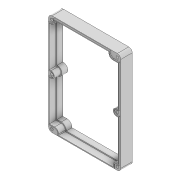
# Autodesk Inventor part: elektrobox EGI
Saved by Autodesk Inventor 2020.3 (Build 243373000, 373)
## iProperties
Created: 2020-12-12
Part Number: elektrobox EGI
Material: Generic
Document SubType Name: Modeling
Designer: Svend
Density: 1 g/cm^3
Appearance: Default
Author: Svend
Autodesk Inventor part; units mm, degrees
ref_plane "YZ Plane" through (0, 0, 0) normal (1, 0, 0) x (0, 1, 0)
ref_plane "XZ Plane" through (0, 0, 0) normal (0, 1, 0) x (-1, 0, 0)
ref_plane "XY Plane" through (0, 0, 0) normal (0, 0, 1) x (1, 0, 0)
sketch "Sketch1" plane through (0, 0, 0) normal (0, 0, 1) x (1, 0, 0)
  line L0 (-54.1322, 76.0214) -> (-53.917, 75.769)
  line L1 (40.9938, 75.769) -> (41.2072, 76.0214)
  line L2 (41.2072, 76.0214) -> (-54.1322, 76.0214)
  line L3 (-54.1322, 76.0214) -> (-54.1322, 72.8159)
  arc A0 (-59.6431, 67.3051) -> (-54.1322, 72.8159) centre (-59.6431, 72.8159) ccw
  line L4 (-59.6431, 67.3051) -> (-62.8486, 67.3051)
  line L5 (-62.8486, 67.3051) -> (-62.8486, -3.4861)
  line L6 (-62.8486, -3.4861) -> (-59.8427, -3.4861)
  arc A1 (-59.8427, -15.1085) -> (-59.8427, -3.4861) centre (-59.8427, -9.2973) ccw
  line L7 (-59.8427, -15.1085) -> (-62.8486, -15.1085)
  line L8 (-62.8486, -15.1085) -> (-62.8486, -85.5495)
  line L9 (-62.8486, -85.5495) -> (-53.6313, -85.5495)
  arc A2 (-46.6155, -92.5632) -> (-53.6313, -85.5495) centre (-53.6303, -92.5642) ccw
  line L10 (-46.6155, -92.5632) -> (-46.6155, -94.8177)
  line L11 (-46.4531, -94.5652) -> (-46.6155, -94.8177)
  line L12 (-46.6155, -94.8177) -> (48.673, -94.8177)
  line L13 (48.673, -94.8177) -> (48.4577, -94.5652)
  line L14 (55.9235, -91.1346) -> (55.9235, -93.5398)
  line L15 (55.9235, -93.5398) -> (53.5184, -93.5398)
  line L16 (53.5184, -93.5398) -> (53.5184, -91.1346)
  line L17 (53.5184, -91.1346) -> (55.9235, -91.1346)
  line L18 (53.5184, -10.8013) -> (53.5184, -8.3961)
  line L19 (53.5184, -8.3961) -> (55.9235, -8.3961)
  line L20 (55.9235, -8.3961) -> (55.9235, -10.8013)
  line L21 (55.9235, -10.8013) -> (53.5184, -10.8013)
  line L22 (55.9235, 74.3443) -> (55.9235, 71.9392)
  line L23 (55.9235, 71.9392) -> (53.5184, 71.9392)
  line L24 (53.5184, 71.9392) -> (53.5184, 74.3443)
  line L25 (53.5184, 74.3443) -> (55.9235, 74.3443)
  line L26 (-60.9816, 71.9392) -> (-60.9816, 74.3443)
  line L27 (-60.9816, 74.3443) -> (-58.5765, 74.3443)
  line L28 (-58.5765, 74.3443) -> (-58.5765, 71.9392)
  line L29 (-58.5765, 71.9392) -> (-60.9816, 71.9392)
  line L30 (-58.5765, -8.3961) -> (-58.5765, -10.8013)
  line L31 (-58.5765, -10.8013) -> (-60.9816, -10.8013)
  line L32 (-60.9816, -10.8013) -> (-60.9816, -8.3961)
  line L33 (-60.9816, -8.3961) -> (-58.5765, -8.3961)
  line L34 (-60.9816, -93.5398) -> (-60.9816, -91.1346)
  line L35 (-60.9816, -91.1346) -> (-58.5765, -91.1346)
  line L36 (-58.5765, -91.1346) -> (-58.5765, -93.5398)
  line L37 (-58.5765, -93.5398) -> (-60.9816, -93.5398)
  arc A3 (60.495, 73.0155) -> (54.4883, 79.0273) centre (54.4883, 73.0207) ccw
  line L38 (60.495, 73.0155) -> (60.495, -91.7609)
  arc A4 (54.4883, -97.7727) -> (60.495, -91.7609) centre (54.4883, -91.766) ccw
  line L39 (54.4883, -97.7727) -> (-59.5464, -97.7727)
  arc A5 (-65.5531, -91.7609) -> (-59.5464, -97.7727) centre (-59.5464, -91.766) ccw
  line L40 (-65.5531, -91.7609) -> (-65.5531, 73.0155)
  arc A6 (-59.5413, 79.0273) -> (-65.5531, 73.0155) centre (-59.5464, 73.0207) ccw
  line L41 (-59.5413, 79.0273) -> (54.4883, 79.0273)
  line L42 (-62.6979, -85.3244) -> (-53.4669, -85.3244)
  arc A7 (-46.4531, -92.3382) -> (-53.4669, -85.3244) centre (-53.462, -92.3333) ccw
  line L43 (-46.4531, -92.3382) -> (-46.4531, -94.5652)
  line L44 (-46.4531, -94.5652) -> (48.4577, -94.5652)
  line L45 (48.4577, -94.5652) -> (48.4577, -91.3362)
  arc A8 (53.9685, -85.8254) -> (48.4577, -91.3362) centre (53.9674, -91.3351) ccw
  line L46 (53.9685, -85.8254) -> (57.2386, -85.8254)
  line L47 (-62.6979, -3.2102) -> (-59.9542, -3.2102)
  arc A9 (-59.9542, -15.5841) -> (-59.9542, -3.2102) centre (-59.9532, -9.3971) ccw
  line L48 (-59.9542, -15.5841) -> (-62.6979, -15.5841)
  line L49 (57.2386, 66.5282) -> (48.0076, 66.5282)
  arc A10 (40.9938, 73.542) -> (48.0076, 66.5282) centre (48.0094, 73.5438) ccw
  line L50 (40.9938, 73.542) -> (40.9938, 75.769)
  line L51 (40.9938, 75.769) -> (-53.917, 75.769)
  line L52 (-53.917, 75.769) -> (-53.917, 72.54)
  arc A11 (-59.4278, 67.0292) -> (-53.917, 72.54) centre (-59.4299, 72.5421) ccw
  line L53 (-59.4278, 67.0292) -> (-62.6979, 67.0292)
  line L54 (57.2386, -15.6858) -> (54.5204, -15.6858)
  arc A12 (54.5204, -3.3609) -> (54.5204, -15.6858) centre (54.5204, -9.5234) ccw
  line L55 (54.5204, -3.3609) -> (57.2386, -3.3609)
  line L56 (36.348, -56.4885) -> (36.348, -54.1343)
  line L57 (36.348, -54.1343) -> (38.7022, -54.1343)
  line L58 (38.7022, -54.1343) -> (38.7022, -56.4885)
  line L59 (38.7022, -56.4885) -> (36.348, -56.4885)
  line L60 (-57.7879, -78.3107) -> (-57.7879, -75.9545)
  line L61 (-57.7879, -75.9545) -> (-55.4336, -75.9545)
  line L62 (-55.4336, -75.9545) -> (-55.4336, -78.3107)
  line L63 (-55.4336, -78.3107) -> (-57.7879, -78.3107)
  line L64 (-57.7879, -25.5039) -> (-57.7879, -23.1497)
  line L65 (-57.7879, -23.1497) -> (-55.4336, -23.1497)
  line L66 (-55.4336, -23.1497) -> (-55.4336, -25.5039)
  line L67 (-55.4336, -25.5039) -> (-57.7879, -25.5039)
  line L68 (-57.7879, 4.3554) -> (-57.7879, 6.7097)
  line L69 (-57.7879, 6.7097) -> (-55.4336, 6.7097)
  line L70 (-55.4336, 6.7097) -> (-55.4336, 4.3554)
  line L71 (-55.4336, 4.3554) -> (-57.7879, 4.3554)
  line L72 (-43.911, 35.7393) -> (-43.911, 38.0955)
  line L73 (-43.911, 38.0955) -> (-41.5568, 38.0955)
  line L74 (-41.5568, 38.0955) -> (-41.5568, 35.7393)
  line L75 (-41.5568, 35.7393) -> (-43.911, 35.7393)
  line L76 (-57.7879, 57.1602) -> (-57.7879, 59.5144)
  line L77 (-57.7879, 59.5144) -> (-55.4336, 59.5144)
  line L78 (-55.4336, 59.5144) -> (-55.4336, 57.1602)
  line L79 (-55.4336, 57.1602) -> (-57.7879, 57.1602)
  line L80 (52.3795, 57.1602) -> (50.0252, 57.1602)
  line L81 (50.0252, 57.1602) -> (50.0252, 59.5144)
  line L82 (50.0252, 59.5144) -> (52.3795, 59.5144)
  line L83 (52.3795, 59.5144) -> (52.3795, 57.1602)
  line L84 (36.348, 35.7393) -> (36.348, 38.0955)
  line L85 (36.348, 38.0955) -> (38.7022, 38.0955)
  line L86 (38.7022, 38.0955) -> (38.7022, 35.7393)
  line L87 (38.7022, 35.7393) -> (36.348, 35.7393)
  line L88 (50.0252, 4.3554) -> (50.0252, 6.7097)
  line L89 (50.0252, 6.7097) -> (52.3795, 6.7097)
  line L90 (52.3795, 6.7097) -> (52.3795, 4.3554)
  line L91 (52.3795, 4.3554) -> (50.0252, 4.3554)
  line L92 (50.0252, -25.5039) -> (50.0252, -23.1497)
  line L93 (50.0252, -23.1497) -> (52.3795, -23.1497)
  line L94 (52.3795, -23.1497) -> (52.3795, -25.5039)
  line L95 (52.3795, -25.5039) -> (50.0252, -25.5039)
  line L96 (-43.911, -56.4885) -> (-43.911, -54.1343)
  line L97 (-43.911, -54.1343) -> (-41.5568, -54.1343)
  line L98 (-41.5568, -54.1343) -> (-41.5568, -56.4885)
  line L99 (-41.5568, -56.4885) -> (-43.911, -56.4885)
  line L100 (50.0252, -78.3107) -> (50.0252, -75.9545)
  line L101 (50.0252, -75.9545) -> (52.3795, -75.9545)
  line L102 (52.3795, -75.9545) -> (52.3795, -78.3107)
  line L103 (52.3795, -78.3107) -> (50.0252, -78.3107)
  line L104 (-62.6979, -34.6723) -> (-62.6979, -59.7234)
  line L105 (-62.6979, -61.2264) -> (-62.6979, -64.0307)
  line L106 (-62.6979, -65.5336) -> (-62.6979, -85.3244)
  line L107 (-62.6979, -85.3244) -> (-62.8486, -85.5495)
  line L108 (-62.6979, -28.8621) -> (-62.6979, -15.5841)
  line L109 (-62.6979, -15.5841) -> (-62.8486, -15.1085)
  line L110 (-62.6979, -30.365) -> (-62.6979, -33.1694)
  line L111 (-62.6979, 13.923) -> (-62.6979, 11.1187)
  line L112 (-62.6979, 9.6158) -> (-62.6979, -3.2102)
  line L113 (-62.6979, -3.2102) -> (-62.8486, -3.4861)
  line L114 (-62.8486, 67.3051) -> (-62.6979, 67.0292)
  line L115 (-62.6979, 67.0292) -> (-62.6979, 46.2873)
  line L116 (-62.6979, 44.7844) -> (-62.6979, 41.98)
  line L117 (-62.6979, 40.4771) -> (-62.6979, 15.426)
  line L118 (-62.8251, -64.0307) -> (-61.2712, -64.0307)
  line L119 (-61.2712, -64.0307) -> (-61.146, -64.0307)
  line L120 (-61.146, -64.0307) -> (-61.146, -65.5336)
  line L121 (-61.146, -65.5336) -> (-61.2712, -65.5336)
  line L122 (-61.2712, -65.5336) -> (-62.8251, -65.5336)
  line L123 (-62.8251, -65.5336) -> (-62.8251, -64.0307)
  line L124 (-61.2712, -64.0307) -> (-61.2712, -65.5336)
  line L125 (-61.2712, 11.1187) -> (-61.146, 11.1187)
  line L126 (-61.146, 11.1187) -> (-61.146, 9.6158)
  line L127 (-61.146, 9.6158) -> (-61.2712, 9.6158)
  line L128 (-61.2712, 9.6158) -> (-62.8251, 9.6158)
  line L129 (-62.8251, 9.6158) -> (-62.8251, 11.1187)
  line L130 (-62.8251, 11.1187) -> (-61.2712, 11.1187)
  line L131 (-61.2712, 11.1187) -> (-61.2712, 9.6158)
  line L132 (-61.2712, 41.98) -> (-61.146, 41.98)
  line L133 (-61.146, 41.98) -> (-61.146, 40.4771)
  line L134 (-61.146, 40.4771) -> (-61.2712, 40.4771)
  line L135 (-61.2712, 40.4771) -> (-62.8251, 40.4771)
  line L136 (-62.8251, 40.4771) -> (-62.8251, 41.98)
  line L137 (-62.8251, 41.98) -> (-61.2712, 41.98)
  line L138 (-61.2712, 41.98) -> (-61.2712, 40.4771)
  line L139 (-61.2712, -28.8621) -> (-61.146, -28.8621)
  line L140 (-61.146, -28.8621) -> (-61.146, -30.365)
  line L141 (-61.146, -30.365) -> (-61.2712, -30.365)
  line L142 (-61.2712, -30.365) -> (-62.8251, -30.365)
  line L143 (-62.8251, -30.365) -> (-62.8251, -28.8621)
  line L144 (-62.8251, -28.8621) -> (-61.2712, -28.8621)
  line L145 (-61.2712, -28.8621) -> (-61.2712, -30.365)
  line L146 (-61.2712, -59.7234) -> (-61.146, -59.7234)
  line L147 (-61.146, -59.7234) -> (-61.146, -61.2264)
  line L148 (-61.146, -61.2264) -> (-61.2712, -61.2264)
  line L149 (-61.2712, -61.2264) -> (-62.8251, -61.2264)
  line L150 (-62.8251, -61.2264) -> (-62.8251, -59.7234)
  line L151 (-62.8251, -59.7234) -> (-61.2712, -59.7234)
  line L152 (-61.2712, -59.7234) -> (-61.2712, -61.2264)
  line L153 (-61.2712, 46.2873) -> (-61.146, 46.2873)
  line L154 (-61.146, 46.2873) -> (-61.146, 44.7844)
  line L155 (-61.146, 44.7844) -> (-61.2712, 44.7844)
  line L156 (-61.2712, 44.7844) -> (-62.8251, 44.7844)
  line L157 (-62.8251, 44.7844) -> (-62.8251, 46.2873)
  line L158 (-62.8251, 46.2873) -> (-61.2712, 46.2873)
  line L159 (-61.2712, 46.2873) -> (-61.2712, 44.7844)
  line L160 (-61.2712, 15.426) -> (-61.146, 15.426)
  line L161 (-61.146, 15.426) -> (-61.146, 13.923)
  line L162 (-61.146, 13.923) -> (-61.2712, 13.923)
  line L163 (-61.2712, 13.923) -> (-62.8251, 13.923)
  line L164 (-62.8251, 13.923) -> (-62.8251, 15.426)
  line L165 (-62.8251, 15.426) -> (-61.2712, 15.426)
  line L166 (-61.2712, 15.426) -> (-61.2712, 13.923)
  line L167 (-61.2712, -33.1694) -> (-61.146, -33.1694)
  line L168 (-61.146, -33.1694) -> (-61.146, -34.6723)
  line L169 (-61.146, -34.6723) -> (-61.2712, -34.6723)
  line L170 (-61.2712, -34.6723) -> (-62.8251, -34.6723)
  line L171 (-62.8251, -34.6723) -> (-62.8251, -33.1694)
  line L172 (-62.8251, -33.1694) -> (-61.2712, -33.1694)
  line L173 (-61.2712, -33.1694) -> (-61.2712, -34.6723)
  line L174 (57.2386, 11.2674) -> (57.2386, 14.0737)
  line L175 (57.2386, 15.5767) -> (57.2386, 40.6258)
  line L176 (57.2386, 42.1307) -> (57.2386, 44.935)
  line L177 (57.2386, 46.438) -> (57.2386, 66.5282)
  line L178 (57.2386, 66.5282) -> (57.3893, 66.7532)
  line L179 (57.2386, 9.7645) -> (57.2386, -3.3609)
  line L180 (57.2386, -3.3609) -> (57.3893, -3.5859)
  line L181 (57.2386, -28.6605) -> (57.2386, -15.6858)
  line L182 (57.2386, -15.6858) -> (57.3893, -15.2083)
  line L183 (57.2386, -65.334) -> (57.2386, -85.8254)
  line L184 (57.2386, -85.8254) -> (57.3893, -86.0505)
  line L185 (57.3893, -86.0505) -> (54.1838, -86.0505)
  arc A13 (54.1838, -86.0505) -> (48.673, -91.5613) centre (54.1838, -91.5613) ccw
  line L186 (48.673, -91.5613) -> (48.673, -94.8177)
  line L187 (57.2386, -63.8311) -> (57.2386, -61.0248)
  line L188 (57.2386, -59.5218) -> (57.2386, -34.4727)
  line L189 (57.2386, -32.9698) -> (57.2386, -30.1635)
  line L190 (57.3658, 44.935) -> (55.8629, 44.935)
  line L191 (55.8629, 44.935) -> (55.7357, 44.935)
  line L192 (55.7357, 44.935) -> (55.7357, 46.438)
  line L193 (55.7357, 46.438) -> (55.8629, 46.438)
  line L194 (55.8629, 46.438) -> (57.3658, 46.438)
  line L195 (57.3658, 46.438) -> (57.3658, 44.935)
  line L196 (55.8629, 44.935) -> (55.8629, 46.438)
  line L197 (55.8629, -34.4727) -> (55.7357, -34.4727)
  line L198 (55.7357, -34.4727) -> (55.7357, -32.9698)
  line L199 (55.7357, -32.9698) -> (55.8629, -32.9698)
  line L200 (55.8629, -32.9698) -> (57.3658, -32.9698)
  line L201 (57.3658, -32.9698) -> (57.3658, -34.4727)
  line L202 (57.3658, -34.4727) -> (55.8629, -34.4727)
  line L203 (55.8629, -34.4727) -> (55.8629, -32.9698)
  line L204 (55.8629, -65.334) -> (55.7357, -65.334)
  line L205 (55.7357, -65.334) -> (55.7357, -63.8311)
  line L206 (55.7357, -63.8311) -> (55.8629, -63.8311)
  line L207 (55.8629, -63.8311) -> (57.3658, -63.8311)
  line L208 (57.3658, -63.8311) -> (57.3658, -65.334)
  line L209 (57.3658, -65.334) -> (55.8629, -65.334)
  line L210 (55.8629, -65.334) -> (55.8629, -63.8311)
  line L211 (55.8629, 14.0737) -> (55.7357, 14.0737)
  line L212 (55.7357, 14.0737) -> (55.7357, 15.5767)
  line L213 (55.7357, 15.5767) -> (55.8629, 15.5767)
  line L214 (55.8629, 15.5767) -> (57.3658, 15.5767)
  line L215 (57.3658, 15.5767) -> (57.3658, 14.0737)
  line L216 (57.3658, 14.0737) -> (55.8629, 14.0737)
  line L217 (55.8629, 14.0737) -> (55.8629, 15.5767)
  line L218 (55.8629, 40.6258) -> (55.7357, 40.6258)
  line L219 (55.7357, 40.6258) -> (55.7357, 42.1307)
  line L220 (55.7357, 42.1307) -> (55.8629, 42.1307)
  line L221 (55.8629, 42.1307) -> (57.3658, 42.1307)
  line L222 (57.3658, 42.1307) -> (57.3658, 40.6258)
  line L223 (57.3658, 40.6258) -> (55.8629, 40.6258)
  line L224 (55.8629, 40.6258) -> (55.8629, 42.1307)
  circle A14 centre (-51.8573, -91.8108) radius 2.3807
  line L225 (55.8629, 9.7645) -> (55.7357, 9.7645)
  line L226 (55.7357, 9.7645) -> (55.7357, 11.2674)
  line L227 (55.7357, 11.2674) -> (55.8629, 11.2674)
  line L228 (55.8629, 11.2674) -> (57.3658, 11.2674)
  line L229 (57.3658, 11.2674) -> (57.3658, 9.7645)
  line L230 (57.3658, 9.7645) -> (55.8629, 9.7645)
  line L231 (55.8629, 9.7645) -> (55.8629, 11.2674)
  circle A15 centre (46.1279, 73.0674) radius 2.3807
  line L232 (55.8629, -61.0248) -> (55.7357, -61.0248)
  line L233 (55.7357, -61.0248) -> (55.7357, -59.5218)
  line L234 (55.7357, -59.5218) -> (55.8629, -59.5218)
  line L235 (55.8629, -59.5218) -> (57.3658, -59.5218)
  line L236 (57.3658, -59.5218) -> (57.3658, -61.0248)
  line L237 (57.3658, -61.0248) -> (55.8629, -61.0248)
  line L238 (55.8629, -61.0248) -> (55.8629, -59.5218)
  line L239 (55.8629, -30.1635) -> (55.7357, -30.1635)
  line L240 (55.7357, -30.1635) -> (55.7357, -28.6605)
  line L241 (55.7357, -28.6605) -> (55.8629, -28.6605)
  line L242 (55.8629, -28.6605) -> (57.3658, -28.6605)
  line L243 (57.3658, -28.6605) -> (57.3658, -30.1635)
  line L244 (57.3658, -30.1635) -> (55.8629, -30.1635)
  line L245 (55.8629, -30.1635) -> (55.8629, -28.6605)
  circle A16 centre (37.5251, -55.3114) radius 3.0303
  circle A17 centre (-56.6127, -77.1316) radius 3.0304
  circle A18 centre (-56.6127, -24.3268) radius 3.0303
  circle A19 centre (-56.6127, 5.5326) radius 3.0303
  circle A20 centre (-42.7339, 36.9184) radius 3.0303
  circle A21 centre (-56.6127, 58.3373) radius 3.0303
  circle A22 centre (51.2024, 58.3373) radius 3.0303
  circle A23 centre (37.5251, 36.9184) radius 3.0303
  circle A24 centre (51.2024, 5.5326) radius 3.0303
  circle A25 centre (51.2024, -24.3268) radius 3.0303
  line L246 (41.2072, 76.0214) -> (41.2052, 73.768)
  arc A26 (41.2052, 73.768) -> (48.2209, 66.7532) centre (48.2204, 73.7685) ccw
  line L247 (48.2209, 66.7532) -> (57.3893, 66.7532)
  line L248 (57.3893, 66.7532) -> (57.3893, -3.5859)
  line L249 (57.3893, -3.5859) -> (54.4832, -3.5859)
  arc A27 (54.4832, -3.5859) -> (54.4832, -15.2083) centre (54.4822, -9.3971) ccw
  line L250 (54.4832, -15.2083) -> (57.3893, -15.2083)
  line L251 (57.3893, -15.2083) -> (57.3893, -86.0505)
  arc A28 (-47.9734, -92.4233) -> (-49.5938, -88.595) centre (-51.8574, -91.8102) ccw
  arc A29 (-47.9698, -92.5632) -> (-47.9734, -92.4233) centre (-53.6728, -92.6423) ccw
  line L252 (-47.9698, -92.5632) -> (-47.9698, -96.1699)
  line L253 (-47.9698, -96.1699) -> (50.0252, -96.1699)
  line L254 (50.0252, -96.1699) -> (50.0252, -91.5603)
  arc A30 (54.1838, -87.4027) -> (50.0252, -91.5603) centre (54.1833, -91.5608) ccw
  line L255 (54.1838, -87.4027) -> (58.7416, -87.4027)
  line L256 (58.7416, -87.4027) -> (58.7416, -13.8561)
  line L257 (58.7416, -13.8561) -> (54.4832, -13.8561)
  arc A31 (54.4832, -4.9382) -> (54.4832, -13.8561) centre (54.4842, -9.3971) ccw
  line L258 (54.4832, -4.9382) -> (58.7416, -4.9382)
  line L259 (58.7416, -4.9382) -> (58.7416, 68.1055)
  line L260 (58.7416, 68.1055) -> (48.2209, 68.1055)
  arc A32 (44.535, 69.4712) -> (48.2209, 68.1055) centre (48.2231, 73.7684) ccw
  arc A33 (42.5597, 74.7204) -> (44.535, 69.4712) centre (46.1281, 73.0669) ccw
  circle A34 centre (-42.7339, -55.3114) radius 3.0303
  circle A35 centre (51.2024, -77.1316) radius 3.0304
  arc A36 (44.5353, 69.4718) -> (42.5594, 74.72) centre (46.1276, 73.0674) ccw
  line L261 (42.5594, 74.72) -> (42.5594, 77.3756)
  line L262 (42.5594, 77.3756) -> (-55.4845, 77.3756)
  line L263 (-55.4845, 77.3756) -> (-55.4845, 72.8159)
  arc A37 (-59.6431, 68.6574) -> (-55.4845, 72.8159) centre (-59.643, 72.8159) ccw
  line L264 (-59.6431, 68.6574) -> (-64.2008, 68.6574)
  line L265 (-64.2008, 68.6574) -> (-64.2008, -4.8384)
  line L266 (-64.2008, -4.8384) -> (-59.8427, -4.8384)
  arc A38 (-59.8427, -13.7563) -> (-59.8427, -4.8384) centre (-59.8436, -9.2973) ccw
  line L267 (-59.8427, -13.7563) -> (-64.2008, -13.7563)
  line L268 (-64.2008, -13.7563) -> (-64.2008, -86.9017)
  line L269 (-64.2008, -86.9017) -> (-53.6313, -86.9017)
  arc A39 (-49.5945, -88.5951) -> (-53.6313, -86.9017) centre (-53.6317, -92.5611) ccw
  arc A40 (-49.5945, -88.5951) -> (-47.9728, -92.4236) centre (-51.8575, -91.8114) ccw
  line L270 (-59.7781, 76.3463) -> (-59.7781, 69.9353)
  line L271 (-56.5726, 73.1408) -> (-62.9855, 73.1408)
  line L272 (54.72, 76.3463) -> (54.72, 69.9353)
  line L273 (57.9275, 73.1408) -> (51.5145, 73.1408)
  line L274 (-59.7781, -6.3922) -> (-59.7781, -12.8052)
  line L275 (-56.5726, -9.5977) -> (-62.9855, -9.5977)
  line L276 (54.72, -6.3922) -> (54.72, -12.8052)
  line L277 (57.9275, -9.5977) -> (51.5145, -9.5977)
  line L278 (54.72, -89.1307) -> (54.72, -95.5437)
  line L279 (57.9275, -92.3362) -> (51.5145, -92.3362)
  line L280 (-59.7781, -89.1307) -> (-59.7781, -95.5437)
  line L281 (-56.5726, -92.3362) -> (-62.9855, -92.3362)
  line L282 (46.1289, 79.0019) -> (46.1289, 67.129)
  line L283 (52.0644, 73.0664) -> (40.1915, 73.0664)
  line L284 (51.2014, 63.3716) -> (51.2014, 53.3011)
  line L285 (56.2366, 58.3363) -> (46.1661, 58.3363)
  line L286 (-51.8563, -85.8743) -> (-51.8563, -97.7472)
  line L287 (-45.9189, -91.8098) -> (-57.7918, -91.8098)
  line L288 (37.5241, 41.9526) -> (37.5241, 31.8821)
  line L289 (42.5594, 36.9174) -> (32.4908, 36.9174)
  line L290 (-42.7329, 41.9526) -> (-42.7329, 31.8821)
  line L291 (-37.6996, 36.9174) -> (-47.7682, 36.9174)
  line L292 (-56.6117, 63.3716) -> (-56.6117, 53.3011)
  line L293 (-51.5764, 58.3363) -> (-61.645, 58.3363)
  line L294 (-56.6117, 10.5668) -> (-56.6117, 0.4963)
  line L295 (-51.5764, 5.5316) -> (-61.645, 5.5316)
  line L296 (51.2014, 10.5668) -> (51.2014, 0.4963)
  line L297 (56.2366, 5.5316) -> (46.1661, 5.5316)
  line L298 (51.2014, -19.2925) -> (51.2014, -29.3611)
  line L299 (56.2366, -24.3278) -> (46.1661, -24.3278)
  line L300 (37.5241, -50.2771) -> (37.5241, -60.3457)
  line L301 (42.5594, -55.3105) -> (32.4908, -55.3105)
  line L302 (51.2014, -72.0973) -> (51.2014, -82.1659)
  line L303 (56.2366, -77.1306) -> (46.1661, -77.1306)
  line L304 (-56.6117, -72.0973) -> (-56.6117, -82.1659)
  line L305 (-51.5764, -77.1306) -> (-61.645, -77.1306)
  line L306 (-42.7329, -50.2771) -> (-42.7329, -60.3457)
  line L307 (-37.6996, -55.3105) -> (-47.7682, -55.3105)
  line L308 (-56.6117, -19.2925) -> (-56.6117, -29.3611)
  line L309 (-51.5764, -24.3278) -> (-61.645, -24.3278)
  line L310 (47.2052, -94.5633) -> (19.1639, -94.5633)
  line L311 (39.7414, 75.769) -> (19.1639, 75.769)
  line L312 (21.1678, -94.5633) -> (21.1678, -91.5574)
  line L313 (21.1678, -91.5574) -> (21.1678, 72.7631)
  line L314 (21.1678, 72.7631) -> (21.1678, 75.769)
  line L315 (21.9721, -91.5574) -> (21.1678, -94.5633)
  line L316 (21.1678, -94.5633) -> (20.3616, -91.5574)
  line L317 (20.3616, 72.7631) -> (21.1678, 75.769)
  line L318 (21.1678, 75.769) -> (21.9721, 72.7631)
  line L319 (-62.6979, -84.07) -> (-62.6979, -64.4514)
  line L320 (57.2386, -84.571) -> (57.2386, -64.4514)
  line L321 (-62.6979, -66.4554) -> (-59.692, -66.4554)
  line L322 (-59.692, -66.4554) -> (54.2327, -66.4554)
  line L323 (54.2327, -66.4554) -> (57.2386, -66.4554)
  line L324 (-59.692, -67.2616) -> (-62.6979, -66.4554)
  line L325 (-62.6979, -66.4554) -> (-59.692, -65.6511)
  line L326 (54.2327, -65.6511) -> (57.2386, -66.4554)
  line L327 (57.2386, -66.4554) -> (54.2327, -67.2616)
  line L328 (46.1289, -49.5002) -> (46.1289, -69.5395)
  line L329 (46.1289, -69.5395) -> (48.6651, -69.5395)
  line L330 (48.6651, -69.5395) -> (51.2014, -69.5395)
  line L331 (51.2014, -69.5395) -> (51.2014, -76.4789)
  line L332 (51.2014, -76.4789) -> (51.2014, -83.4183)
  line L333 (51.2014, -83.4183) -> (52.9607, -83.4183)
  line L334 (52.9607, -83.4183) -> (54.72, -83.4183)
  line L335 (54.72, -83.4183) -> (54.72, -103.4577)
  circle A41 centre (57.2376, 43.5329) radius 6.2378
  line L336 (-0.8402, 73.0664) -> (40.943, 73.0664)
  line L337 (40.943, 73.0664) -> (-0.8402, 73.0664)
  line L338 (-58.2888, 79.0273) -> (3.1677, 79.0273)
  line L339 (1.9681, 82.0332) -> (1.1637, 79.0273)
  line L340 (1.1637, 79.0273) -> (0.3575, 82.0332)
  line L341 (-54.5354, -91.8098) -> (3.1677, -91.8098)
  line L342 (1.1637, 73.0664) -> (1.1637, 70.0605)
  line L343 (1.1637, 70.0605) -> (1.1637, -88.8039)
  line L344 (1.1637, -88.8039) -> (1.1637, -91.8098)
  line L345 (1.9681, -88.8039) -> (1.1637, -91.8098)
  line L346 (1.1637, -91.8098) -> (0.3575, -88.8039)
  line L347 (-29.6976, 61.8413) -> (-51.414, 69.6554)
  line L348 (-51.414, 69.6554) -> (-54.2418, 70.673)
  line L349 (-54.2418, 70.673) -> (-51.142, 70.4128)
  line L350 (-59.4278, 72.54) -> (-54.2418, 70.673)
  line L351 (-54.2418, 70.673) -> (-51.686, 68.8981)
  line L352 (27.8039, 63.3266) -> (39.0662, 69.0194)
  line L353 (39.0662, 69.0194) -> (41.7473, 70.3775)
  line L354 (41.7473, 70.3775) -> (39.4283, 68.3012)
  line L355 (48.0076, 73.542) -> (41.7473, 70.3775)
  line L356 (41.7473, 70.3775) -> (38.7022, 69.7396)
  line L357 (-37.4393, -76.3459) -> (-46.3729, -85.2598)
  line L358 (-46.3729, -85.2598) -> (-48.5021, -87.3831)
  line L359 (-48.5021, -87.3831) -> (-46.9424, -84.6884)
  line L360 (-53.4669, -92.3362) -> (-48.5021, -87.3831)
  line L361 (-48.5021, -87.3831) -> (-45.8054, -85.8293)
  line L362 (30.5554, -79.342) -> (46.3892, -87.4516)
  line L363 (46.3892, -87.4516) -> (49.0644, -88.8215)
  line L364 (49.0644, -88.8215) -> (46.0213, -88.1679)
  line L365 (53.9685, -91.3343) -> (49.0644, -88.8215)
  line L366 (49.0644, -88.8215) -> (46.7551, -86.7354)
  line L367 (-53.7643, -8.1457) -> (-53.7643, 2.5002)
  line L368 (48.3559, -8.2709) -> (48.3559, 2.5002)
  line L369 (-53.7643, 0.4963) -> (-50.7584, 0.4963)
  line L370 (-50.7584, 0.4963) -> (45.35, 0.4963)
  line L371 (45.35, 0.4963) -> (48.3559, 0.4963)
  line L372 (-50.7584, -0.308) -> (-53.7643, 0.4963)
  line L373 (-53.7643, 0.4963) -> (-50.7584, 1.3026)
  line L374 (45.35, 1.3026) -> (48.3559, 0.4963)
  line L375 (48.3559, 0.4963) -> (45.35, -0.308)
  point P0 (-17.5057, 1.7531)
  point P1 (-22.7014, -65.1985)
  point P2 (-0.0931, -21.271)
  point P3 (19.913, -16.4667)
  point P4 (-42.4594, 67.7678)
  point P5 (27.9233, 64.7904)
  point P6 (-44.5862, -81.706)
  point P7 (31.8111, -78.5747)
  point P8 (-49.667, -88.5453)
  point P9 (-49.6555, -88.5339)
  point P10 (57.3893, 49.7689)
  point P11 (58.7416, 49.5867)
  point P12 (58.7416, 37.4791)
  point P13 (57.3893, 37.2969)
  dimension "d3" = 176.8
  constraints: 752 end point, 64 point on line, 54 point on circle, 42 centre point, 8 other
  measures "d3" distance between parallel lines of L39 L338
extrude "Extrusion1" add sketch "Sketch1" along normal blind 20 contours L3 A0 L350 A37 L263 L262 L261 A33 L283 A26 L246 L2 | A0 L4 L5 L6 A1 L7 L8 L9 A2 L360 A39 L269 L268 L267 A38 L266 L265 L264 A37 L350 | L283 A33 L355 A26 | A37 L264 L265 L266 A38 L267 L268 L269 A39 L286 A40 A29 L252 L253 L254 A30 L365 L17 L16 L15 L278 L335 A4 L39 A5 L40 A6 L41 A3 L38 A41 L259 L260 A32 L282 A36 L261 L262 L263 | L355 A33 A32 L260 L259 A41 L248 L247 A26 | L283 A15 L355 A33 | A33 A36 L282 A15 L283 | L355 A15 L282 A36 A33 | L283 L282 L355 A15 | A15 L282 L283 | A36 L282 A32 | L355 L282 A15 | A36 L283 A15 L282 | A15 L283 L282 | L283 L355 L282 | A41 L259 L248 | L282 A15 L283 A36 | L282 L355 L283 A15 | A41 L259 L258 A31 L257 L256 L255 L335 L185 L251 L250 A27 L249 L248 | A41 L38 L259 | A41 L38 A4 L335 L278 L15 L14 L17 L255 L256 L257 A31 L258 L259 | A2 L287 A28 A39 L360 | L12 L186 A13 L365 A30 L254 L253 L252 A29 A28 L287 A2 L10 | L360 A40 L286 A39 | L287 A14 L360 A40 A28 | A28 A40 L286 A14 L287 | L360 A14 L286 A40 | L286 A14 L287 A40 | A13 L185 L335 L255 A30 L365 | L287 L286 L360 A14 | A14 L286 L287 | L360 L286 A14 | L287 A14 L286 A40 | L286 L360 L287 A14 | A30 L255 L335 L278 L17 L365 | A14 L287 L286 | L287 L360 L286
sketch "Sketch2" plane through (0, 0, 20) normal (0, 0, 1) x (1, 0, 0)
  arc A0 (60.495, 73.0155) -> (54.4883, 79.0273) centre (54.4883, 73.0207) ccw projected
  line L0 (54.4883, 79.0273) -> (-59.5413, 79.0273) projected
  arc A1 (-59.5413, 79.0273) -> (-65.5531, 73.0155) centre (-59.5464, 73.0207) ccw projected
  line L1 (-65.5531, 73.0155) -> (-65.5531, -91.7609) projected
  arc A2 (-65.5531, -91.7609) -> (-59.5464, -97.7727) centre (-59.5464, -91.766) ccw projected
  line L2 (-59.5464, -97.7727) -> (54.4883, -97.7727) projected
  arc A3 (54.4883, -97.7727) -> (60.495, -91.7609) centre (54.4883, -91.766) ccw projected
  line L3 (60.495, -91.7609) -> (60.495, 73.0155) projected
  line L4 (-49.667, -88.5453) -> (-49.6555, -88.5339) projected
  arc A4 (-49.5945, -88.5951) -> (-49.6555, -88.5339) centre (-53.6317, -92.5611) ccw projected
  arc A5 (-49.5945, -88.5951) -> (-49.667, -88.5453) centre (-51.8575, -91.8114) ccw projected
  arc A6 (-46.6155, -92.5632) -> (-53.6313, -85.5495) centre (-53.6303, -92.5642) ccw projected
  line L5 (-53.6313, -85.5495) -> (-62.8486, -85.5495) projected
  line L6 (-62.8486, -85.5495) -> (-62.8486, -15.1085) projected
  line L7 (-62.8486, -15.1085) -> (-59.8427, -15.1085) projected
  arc A7 (-59.8427, -15.1085) -> (-59.8427, -3.4861) centre (-59.8427, -9.2973) ccw projected
  line L8 (-59.8427, -3.4861) -> (-62.8486, -3.4861) projected
  line L9 (-62.8486, -3.4861) -> (-62.8486, 67.3051) projected
  line L10 (-62.8486, 67.3051) -> (-59.6431, 67.3051) projected
  arc A8 (-59.6431, 67.3051) -> (-54.1322, 72.8159) centre (-59.6431, 72.8159) ccw projected
  line L11 (-54.1322, 72.8159) -> (-54.1322, 76.0214) projected
  line L12 (-54.1322, 76.0214) -> (41.2072, 76.0214) projected
  line L13 (41.2072, 76.0214) -> (41.2052, 73.768) projected
  arc A9 (41.2052, 73.768) -> (48.2209, 66.7532) centre (48.2204, 73.7685) ccw projected
  line L14 (48.2209, 66.7532) -> (57.3893, 66.7532) projected
  line L15 (57.3893, 66.7532) -> (57.3893, -3.5859) projected
  line L16 (57.3893, -3.5859) -> (54.4832, -3.5859) projected
  arc A10 (54.4832, -3.5859) -> (54.4832, -15.2083) centre (54.4822, -9.3971) ccw projected
  line L17 (54.4832, -15.2083) -> (57.3893, -15.2083) projected
  line L18 (57.3893, -15.2083) -> (57.3893, -86.0505) projected
  line L19 (57.3893, -86.0505) -> (54.1838, -86.0505) projected
  arc A11 (54.1838, -86.0505) -> (48.673, -91.5613) centre (54.1838, -91.5613) ccw projected
  line L20 (48.673, -91.5613) -> (48.673, -94.8177) projected
  line L21 (48.673, -94.8177) -> (-46.6155, -94.8177) projected
  line L22 (-46.6155, -94.8177) -> (-46.6155, -92.5632) projected
  line L23 (-58.5765, 74.3443) -> (-58.5765, 71.9392) projected
  line L24 (-58.5765, 71.9392) -> (-60.9816, 71.9392) projected
  line L25 (-60.9816, 71.9392) -> (-60.9816, 74.3443) projected
  line L26 (-60.9816, 74.3443) -> (-58.5765, 74.3443) projected
  line L27 (55.9235, -10.8013) -> (53.5184, -10.8013) projected
  line L28 (53.5184, -10.8013) -> (53.5184, -8.3961) projected
  line L29 (53.5184, -8.3961) -> (55.9235, -8.3961) projected
  line L30 (55.9235, -8.3961) -> (55.9235, -10.8013) projected
  line L31 (53.5184, 74.3443) -> (55.9235, 74.3443) projected
  line L32 (55.9235, 74.3443) -> (55.9235, 71.9392) projected
  line L33 (55.9235, 71.9392) -> (53.5184, 71.9392) projected
  line L34 (53.5184, 71.9392) -> (53.5184, 74.3443) projected
  line L35 (-60.9816, -8.3961) -> (-58.5765, -8.3961) projected
  line L36 (-58.5765, -8.3961) -> (-58.5765, -10.8013) projected
  line L37 (-58.5765, -10.8013) -> (-60.9816, -10.8013) projected
  line L38 (-60.9816, -10.8013) -> (-60.9816, -8.3961) projected
  line L39 (-58.5765, -93.5398) -> (-60.9816, -93.5398) projected
  line L40 (-60.9816, -93.5398) -> (-60.9816, -91.1346) projected
  line L41 (-60.9816, -91.1346) -> (-58.5765, -91.1346) projected
  line L42 (-58.5765, -91.1346) -> (-58.5765, -93.5398) projected
  line L43 (53.5184, -91.1346) -> (55.9235, -91.1346) projected
  line L44 (55.9235, -91.1346) -> (55.9235, -93.5398) projected
  line L45 (55.9235, -93.5398) -> (53.5184, -93.5398) projected
  line L46 (53.5184, -93.5398) -> (53.5184, -91.1346) projected
  line L47 (58.8893, 68.2532) -> (48.2204, 68.2532)
  arc A12 (42.7052, 73.7733) -> (48.2204, 68.2532) centre (48.2204, 73.7685) ccw
  line L48 (42.7052, 73.7733) -> (42.7085, 77.5214)
  line L49 (42.7085, 77.5214) -> (-55.6322, 77.5214)
  line L50 (-55.6322, 77.5214) -> (-55.6322, 72.8159)
  arc A13 (-59.6431, 68.8051) -> (-55.6322, 72.8159) centre (-59.6431, 72.8159) ccw
  line L51 (-59.6431, 68.8051) -> (-64.3486, 68.8051)
  line L52 (-64.3486, 68.8051) -> (-64.3486, -4.9861)
  line L53 (-64.3486, -4.9861) -> (-59.8427, -4.9861)
  arc A14 (-59.8427, -13.6085) -> (-59.8427, -4.9861) centre (-59.8427, -9.2973) ccw
  line L54 (-59.8427, -13.6085) -> (-64.3486, -13.6085)
  line L55 (-64.3486, -13.6085) -> (-64.3486, -87.0495)
  line L56 (-64.3486, -87.0495) -> (-53.6303, -87.0495)
  arc A15 (-48.1155, -92.5642) -> (-53.6303, -87.0495) centre (-53.6303, -92.5642) ccw
  line L57 (-48.1155, -92.5642) -> (-48.1155, -96.3177)
  line L58 (-48.1155, -96.3177) -> (50.173, -96.3177)
  line L59 (50.173, -96.3177) -> (50.173, -91.5613)
  arc A16 (54.1838, -87.5505) -> (50.173, -91.5613) centre (54.1838, -91.5613) ccw
  line L60 (54.1838, -87.5505) -> (58.8893, -87.5505)
  line L61 (58.8893, -87.5505) -> (58.8893, -13.7083)
  line L62 (58.8893, -13.7083) -> (54.4822, -13.7083)
  arc A17 (54.4822, -5.0859) -> (54.4822, -13.7083) centre (54.4822, -9.3971) ccw
  line L63 (54.4822, -5.0859) -> (58.8893, -5.0859)
  line L64 (58.8893, -5.0859) -> (58.8893, 68.2532)
  point P0 (0, 0)
  dimension "d4" = 1.5
  constraints: 36 end point, 12 point on circle, 6 centre point, 23 other
  measures "d4" distance between parallel lines of L14 L47
extrude "Extrusion2" add sketch "Sketch2" along normal blind 1.5 contours L64 L63 A17 L62 L61 L60 A16 L59 L58 L57 A15 L56 L55 L54 A14 L53 L52 L51 A13 L50 L49 L48 A12 L47
sketch "Sketch3" plane through (0, 0, 0) normal (0, 0, -1) x (-1, 0, 0)
  arc A0 (-54.4883, 79.0273) -> (-60.495, 73.0155) centre (-54.4883, 73.0207) ccw projected
  line L0 (-60.495, -91.7609) -> (-60.495, 73.0155) projected
  arc A1 (-60.495, -91.7609) -> (-54.4883, -97.7727) centre (-54.4883, -91.766) ccw projected
  line L1 (59.5464, -97.7727) -> (-54.4883, -97.7727) projected
  arc A2 (59.5464, -97.7727) -> (65.5531, -91.7609) centre (59.5464, -91.766) ccw projected
  line L2 (65.5531, 73.0155) -> (65.5531, -91.7609) projected
  arc A3 (65.5531, 73.0155) -> (59.5413, 79.0273) centre (59.5464, 73.0207) ccw projected
  line L3 (-54.4883, 79.0273) -> (59.5413, 79.0273) projected
  line L4 (49.667, -88.5453) -> (49.6555, -88.5339) projected
  arc A4 (49.667, -88.5453) -> (49.5945, -88.5951) centre (51.8575, -91.8114) ccw projected
  arc A5 (49.6555, -88.5339) -> (49.5945, -88.5951) centre (53.6317, -92.5611) ccw projected
  arc A6 (53.6313, -85.5495) -> (46.6155, -92.5632) centre (53.6303, -92.5642) ccw projected
  line L5 (46.6155, -94.8177) -> (46.6155, -92.5632) projected
  line L6 (-48.673, -94.8177) -> (46.6155, -94.8177) projected
  line L7 (-48.673, -91.5613) -> (-48.673, -94.8177) projected
  arc A7 (-48.673, -91.5613) -> (-54.1838, -86.0505) centre (-54.1838, -91.5613) ccw projected
  line L8 (-57.3893, -86.0505) -> (-54.1838, -86.0505) projected
  line L9 (-57.3893, -15.2083) -> (-57.3893, -86.0505) projected
  line L10 (-54.4832, -15.2083) -> (-57.3893, -15.2083) projected
  arc A8 (-54.4832, -15.2083) -> (-54.4832, -3.5859) centre (-54.4822, -9.3971) ccw projected
  line L11 (-57.3893, -3.5859) -> (-54.4832, -3.5859) projected
  line L12 (-57.3893, 66.7532) -> (-57.3893, -3.5859) projected
  line L13 (-48.2209, 66.7532) -> (-57.3893, 66.7532) projected
  arc A9 (-48.2209, 66.7532) -> (-41.2052, 73.768) centre (-48.2204, 73.7685) ccw projected
  line L14 (-41.2072, 76.0214) -> (-41.2052, 73.768) projected
  line L15 (54.1322, 76.0214) -> (-41.2072, 76.0214) projected
  line L16 (54.1322, 72.8159) -> (54.1322, 76.0214) projected
  arc A10 (54.1322, 72.8159) -> (59.6431, 67.3051) centre (59.6431, 72.8159) ccw projected
  line L17 (62.8486, 67.3051) -> (59.6431, 67.3051) projected
  line L18 (62.8486, -3.4861) -> (62.8486, 67.3051) projected
  line L19 (59.8427, -3.4861) -> (62.8486, -3.4861) projected
  arc A11 (59.8427, -3.4861) -> (59.8427, -15.1085) centre (59.8427, -9.2973) ccw projected
  line L20 (62.8486, -15.1085) -> (59.8427, -15.1085) projected
  line L21 (62.8486, -85.5495) -> (62.8486, -15.1085) projected
  line L22 (53.6313, -85.5495) -> (62.8486, -85.5495) projected
  line L23 (58.5765, 74.3443) -> (58.5765, 71.9392) projected
  line L24 (60.9816, 74.3443) -> (58.5765, 74.3443) projected
  line L25 (60.9816, 71.9392) -> (60.9816, 74.3443) projected
  line L26 (58.5765, 71.9392) -> (60.9816, 71.9392) projected
  line L27 (-55.9235, -10.8013) -> (-53.5184, -10.8013) projected
  line L28 (-55.9235, -8.3961) -> (-55.9235, -10.8013) projected
  line L29 (-53.5184, -8.3961) -> (-55.9235, -8.3961) projected
  line L30 (-53.5184, -10.8013) -> (-53.5184, -8.3961) projected
  line L31 (-53.5184, 74.3443) -> (-55.9235, 74.3443) projected
  line L32 (-53.5184, 71.9392) -> (-53.5184, 74.3443) projected
  line L33 (-55.9235, 71.9392) -> (-53.5184, 71.9392) projected
  line L34 (-55.9235, 74.3443) -> (-55.9235, 71.9392) projected
  line L35 (60.9816, -8.3961) -> (58.5765, -8.3961) projected
  line L36 (60.9816, -10.8013) -> (60.9816, -8.3961) projected
  line L37 (58.5765, -10.8013) -> (60.9816, -10.8013) projected
  line L38 (58.5765, -8.3961) -> (58.5765, -10.8013) projected
  line L39 (58.5765, -93.5398) -> (60.9816, -93.5398) projected
  line L40 (58.5765, -91.1346) -> (58.5765, -93.5398) projected
  line L41 (60.9816, -91.1346) -> (58.5765, -91.1346) projected
  line L42 (60.9816, -93.5398) -> (60.9816, -91.1346) projected
  line L43 (-53.5184, -91.1346) -> (-55.9235, -91.1346) projected
  line L44 (-53.5184, -93.5398) -> (-53.5184, -91.1346) projected
  line L45 (-55.9235, -93.5398) -> (-53.5184, -93.5398) projected
  line L46 (-55.9235, -91.1346) -> (-55.9235, -93.5398) projected
  arc A12 (-55.495, -17.0358) -> (-55.495, -1.7585) centre (-54.4822, -9.3971) ccw
  line L47 (-55.495, -17.0358) -> (-55.495, -84.2732)
  arc A13 (-46.905, -92.9234) -> (-55.495, -84.2732) centre (-54.1838, -91.5613) ccw
  line L48 (-46.905, -92.9234) -> (44.7285, -92.9234)
  arc A14 (53.6303, -83.6552) -> (44.7285, -92.9234) centre (53.6303, -92.5642) ccw
  line L49 (53.6303, -83.6552) -> (60.9543, -83.6552)
  line L50 (60.9543, -83.6552) -> (60.9543, -16.9222)
  arc A15 (60.9543, -1.6724) -> (60.9543, -16.9222) centre (59.8427, -9.2973) ccw
  line L51 (60.9543, -1.6724) -> (60.9543, 65.5278)
  arc A16 (52.355, 74.1271) -> (60.9543, 65.5278) centre (59.6431, 72.8159) ccw
  line L52 (52.355, 74.1271) -> (-39.3181, 74.1271)
  arc A17 (-48.2204, 64.8589) -> (-39.3181, 74.1271) centre (-48.2204, 73.7685) ccw
  line L53 (-48.2204, 64.8589) -> (-55.495, 64.8589)
  line L54 (-55.495, 64.8589) -> (-55.495, -1.7585)
  point P0 (0, 0)
  dimension "d7" = 5
  constraints: 16 end point, 12 point on circle, 6 centre point, 13 other
  measures "d7" distance between parallel lines of L0 L54
extrude "Extrusion3" add sketch "Sketch3" against normal blind 10 contours A6 L5 L6 L7 A7 L8 L9 L10 A8 L11 L12 L13 A9 L14 L15 L16 A10 L17 L18 L19 A11 L20 L21 L22
sketch "Sketch4" plane through (0, 0, 0) normal (0, 0, -1) x (-1, 0, 0)
  arc A0 (-46.905, -92.9234) -> (-55.495, -84.2732) centre (-54.1838, -91.5613) ccw projected
  line L0 (-55.495, -84.2732) -> (-55.495, -17.0358) projected
  arc A1 (-55.495, -17.0358) -> (-55.495, -1.7585) centre (-54.4822, -9.3971) ccw projected
  line L1 (-55.495, -1.7585) -> (-55.495, 64.8589) projected
  line L2 (-55.495, 64.8589) -> (-48.2204, 64.8589) projected
  arc A2 (-48.2204, 64.8589) -> (-39.3181, 74.1271) centre (-48.2204, 73.7685) ccw projected
  line L3 (-39.3181, 74.1271) -> (52.355, 74.1271) projected
  arc A3 (52.355, 74.1271) -> (60.9543, 65.5278) centre (59.6431, 72.8159) ccw projected
  line L4 (60.9543, 65.5278) -> (60.9543, -1.6724) projected
  arc A4 (60.9543, -1.6724) -> (60.9543, -16.9222) centre (59.8427, -9.2973) ccw projected
  line L5 (60.9543, -16.9222) -> (60.9543, -83.6552) projected
  line L6 (60.9543, -83.6552) -> (53.6303, -83.6552) projected
  arc A5 (53.6303, -83.6552) -> (44.7285, -92.9234) centre (53.6303, -92.5642) ccw projected
  line L7 (44.7285, -92.9234) -> (-46.905, -92.9234) projected
  arc A6 (-54.4883, 79.0273) -> (-60.495, 73.0155) centre (-54.4883, 73.0207) ccw projected
  line L8 (-60.495, -91.7609) -> (-60.495, 73.0155) projected
  arc A7 (-60.495, -91.7609) -> (-54.4883, -97.7727) centre (-54.4883, -91.766) ccw projected
  line L9 (59.5464, -97.7727) -> (-54.4883, -97.7727) projected
  arc A8 (59.5464, -97.7727) -> (65.5531, -91.7609) centre (59.5464, -91.766) ccw projected
  line L10 (65.5531, 73.0155) -> (65.5531, -91.7609) projected
  arc A9 (65.5531, 73.0155) -> (59.5413, 79.0273) centre (59.5464, 73.0207) ccw projected
  line L11 (-54.4883, 79.0273) -> (59.5413, 79.0273) projected
  line L12 (49.667, -88.5453) -> (49.6555, -88.5339) projected
  arc A10 (49.667, -88.5453) -> (49.5945, -88.5951) centre (51.8575, -91.8114) ccw projected
  arc A11 (49.6555, -88.5339) -> (49.5945, -88.5951) centre (53.6317, -92.5611) ccw projected
  line L13 (58.5765, 74.3443) -> (58.5765, 71.9392) projected
  line L14 (60.9816, 74.3443) -> (58.5765, 74.3443) projected
  line L15 (60.9816, 71.9392) -> (60.9816, 74.3443) projected
  line L16 (58.5765, 71.9392) -> (60.9816, 71.9392) projected
  line L17 (-55.9235, -10.8013) -> (-53.5184, -10.8013) projected
  line L18 (-55.9235, -8.3961) -> (-55.9235, -10.8013) projected
  line L19 (-53.5184, -8.3961) -> (-55.9235, -8.3961) projected
  line L20 (-53.5184, -10.8013) -> (-53.5184, -8.3961) projected
  line L21 (-53.5184, 74.3443) -> (-55.9235, 74.3443) projected
  line L22 (-53.5184, 71.9392) -> (-53.5184, 74.3443) projected
  line L23 (-55.9235, 71.9392) -> (-53.5184, 71.9392) projected
  line L24 (-55.9235, 74.3443) -> (-55.9235, 71.9392) projected
  line L25 (60.9816, -8.3961) -> (58.5765, -8.3961) projected
  line L26 (60.9816, -10.8013) -> (60.9816, -8.3961) projected
  line L27 (58.5765, -10.8013) -> (60.9816, -10.8013) projected
  line L28 (58.5765, -8.3961) -> (58.5765, -10.8013) projected
  line L29 (58.5765, -93.5398) -> (60.9816, -93.5398) projected
  line L30 (58.5765, -91.1346) -> (58.5765, -93.5398) projected
  line L31 (60.9816, -91.1346) -> (58.5765, -91.1346) projected
  line L32 (60.9816, -93.5398) -> (60.9816, -91.1346) projected
  line L33 (-53.5184, -91.1346) -> (-55.9235, -91.1346) projected
  line L34 (-53.5184, -93.5398) -> (-53.5184, -91.1346) projected
  line L35 (-55.9235, -93.5398) -> (-53.5184, -93.5398) projected
  line L36 (-55.9235, -91.1346) -> (-55.9235, -93.5398) projected
  line L37 (-58.8893, -5.0859) -> (-58.8893, 68.2532) projected
  line L38 (-58.8893, 68.2532) -> (-48.2204, 68.2532) projected
  arc A12 (-48.2204, 68.2532) -> (-42.7052, 73.7733) centre (-48.2204, 73.7685) ccw projected
  line L39 (-42.7052, 73.7733) -> (-42.7085, 77.5214) projected
  line L40 (-42.7085, 77.5214) -> (55.6322, 77.5214) projected
  line L41 (55.6322, 77.5214) -> (55.6322, 72.8159) projected
  arc A13 (55.6322, 72.8159) -> (59.6431, 68.8051) centre (59.6431, 72.8159) ccw projected
  line L42 (59.6431, 68.8051) -> (64.3486, 68.8051) projected
  line L43 (64.3486, 68.8051) -> (64.3486, -4.9861) projected
  line L44 (64.3486, -4.9861) -> (59.8427, -4.9861) projected
  arc A14 (59.8427, -4.9861) -> (59.8427, -13.6085) centre (59.8427, -9.2973) ccw projected
  line L45 (59.8427, -13.6085) -> (64.3486, -13.6085) projected
  line L46 (64.3486, -13.6085) -> (64.3486, -87.0495) projected
  line L47 (64.3486, -87.0495) -> (53.6303, -87.0495) projected
  arc A15 (53.6303, -87.0495) -> (48.1155, -92.5642) centre (53.6303, -92.5642) ccw projected
  line L48 (48.1155, -92.5642) -> (48.1155, -96.3177) projected
  line L49 (48.1155, -96.3177) -> (-50.173, -96.3177) projected
  line L50 (-50.173, -96.3177) -> (-50.173, -91.5613) projected
  arc A16 (-50.173, -91.5613) -> (-54.1838, -87.5505) centre (-54.1838, -91.5613) ccw projected
  line L51 (-54.1838, -87.5505) -> (-58.8893, -87.5505) projected
  line L52 (-58.8893, -87.5505) -> (-58.8893, -13.7083) projected
  line L53 (-58.8893, -13.7083) -> (-54.4822, -13.7083) projected
  arc A17 (-54.4822, -13.7083) -> (-54.4822, -5.0859) centre (-54.4822, -9.3971) ccw projected
  line L54 (-54.4822, -5.0859) -> (-58.8893, -5.0859) projected
  arc A18 (53.6313, -85.5495) -> (46.6155, -92.5632) centre (53.6303, -92.5642) ccw projected
  line L55 (53.6313, -85.5495) -> (62.8486, -85.5495) projected
  line L56 (62.8486, -85.5495) -> (62.8486, -15.1085) projected
  line L57 (62.8486, -15.1085) -> (59.8427, -15.1085) projected
  arc A19 (59.8427, -3.4861) -> (59.8427, -15.1085) centre (59.8427, -9.2973) ccw projected
  line L58 (59.8427, -3.4861) -> (62.8486, -3.4861) projected
  line L59 (62.8486, -3.4861) -> (62.8486, 67.3051) projected
  line L60 (62.8486, 67.3051) -> (59.6431, 67.3051) projected
  arc A20 (54.1322, 72.8159) -> (59.6431, 67.3051) centre (59.6431, 72.8159) ccw projected
  line L61 (54.1322, 72.8159) -> (54.1322, 76.0214) projected
  line L62 (54.1322, 76.0214) -> (-41.2072, 76.0214) projected
  line L63 (-41.2072, 76.0214) -> (-41.2052, 73.768) projected
  arc A21 (-48.2209, 66.7532) -> (-41.2052, 73.768) centre (-48.2204, 73.7685) ccw projected
  line L64 (-48.2209, 66.7532) -> (-57.3893, 66.7532) projected
  line L65 (-57.3893, 66.7532) -> (-57.3893, -3.5859) projected
  line L66 (-57.3893, -3.5859) -> (-54.4832, -3.5859) projected
  arc A22 (-54.4832, -15.2083) -> (-54.4832, -3.5859) centre (-54.4822, -9.3971) ccw projected
  line L67 (-54.4832, -15.2083) -> (-57.3893, -15.2083) projected
  line L68 (-57.3893, -15.2083) -> (-57.3893, -86.0505) projected
  line L69 (-57.3893, -86.0505) -> (-54.1838, -86.0505) projected
  arc A23 (-48.673, -91.5613) -> (-54.1838, -86.0505) centre (-54.1838, -91.5613) ccw projected
  line L70 (-48.673, -91.5613) -> (-48.673, -94.8177) projected
  line L71 (-48.673, -94.8177) -> (46.6155, -94.8177) projected
  line L72 (46.6155, -94.8177) -> (46.6155, -92.5632) projected
  arc A24 (49.667, -88.5453) -> (49.5945, -88.5951) centre (51.8575, -91.8114) ccw projected
  line L73 (49.667, -88.5453) -> (49.6555, -88.5339) projected
  arc A25 (49.6555, -88.5339) -> (49.5945, -88.5951) centre (53.6317, -92.5611) ccw projected
  point P0 (0, 0)
extrude "Extrusion4" cut sketch "Sketch4" against normal blind 2.5 contours L37 L38 A12 L39 L40 L41 A13 L42 L43 L44 A14 L45 L46 L47 A15 L48 L49 L50 A16 L51 L52 L53 A17 L54
sketch "Sketch5" plane through (0, 0, 20) normal (0, 0, 1) x (1, 0, 0)
  line L0 (58.8893, -5.0859) -> (54.4822, -5.0859) projected
  arc A0 (54.4822, -5.0859) -> (54.4822, -13.7083) centre (54.4822, -9.3971) ccw projected
  line L1 (54.4822, -13.7083) -> (58.8893, -13.7083) projected
  line L2 (58.8893, -13.7083) -> (58.8893, -87.5505) projected
  line L3 (58.8893, -87.5505) -> (54.1838, -87.5505) projected
  arc A1 (54.1838, -87.5505) -> (50.173, -91.5613) centre (54.1838, -91.5613) ccw projected
  line L4 (50.173, -91.5613) -> (50.173, -96.3177) projected
  line L5 (50.173, -96.3177) -> (-48.1155, -96.3177) projected
  line L6 (-48.1155, -96.3177) -> (-48.1155, -92.5642) projected
  arc A2 (-48.1155, -92.5642) -> (-53.6303, -87.0495) centre (-53.6303, -92.5642) ccw projected
  line L7 (-53.6303, -87.0495) -> (-64.3486, -87.0495) projected
  line L8 (-64.3486, -87.0495) -> (-64.3486, -13.6085) projected
  line L9 (-64.3486, -13.6085) -> (-59.8427, -13.6085) projected
  arc A3 (-59.8427, -13.6085) -> (-59.8427, -4.9861) centre (-59.8427, -9.2973) ccw projected
  line L10 (-59.8427, -4.9861) -> (-64.3486, -4.9861) projected
  line L11 (-64.3486, -4.9861) -> (-64.3486, 68.8051) projected
  line L12 (-64.3486, 68.8051) -> (-59.6431, 68.8051) projected
  arc A4 (-59.6431, 68.8051) -> (-55.6322, 72.8159) centre (-59.6431, 72.8159) ccw projected
  line L13 (-55.6322, 72.8159) -> (-55.6322, 77.5214) projected
  line L14 (-55.6322, 77.5214) -> (42.7085, 77.5214) projected
  line L15 (42.7085, 77.5214) -> (42.7052, 73.7733) projected
  arc A5 (42.7052, 73.7733) -> (48.2204, 68.2532) centre (48.2204, 73.7685) ccw projected
  line L16 (48.2204, 68.2532) -> (58.8893, 68.2532) projected
  line L17 (58.8893, 68.2532) -> (58.8893, -5.0859) projected
  arc A6 (60.495, 73.0155) -> (54.4883, 79.0273) centre (54.4883, 73.0207) ccw projected
  line L18 (54.4883, 79.0273) -> (-59.5413, 79.0273) projected
  arc A7 (-59.5413, 79.0273) -> (-65.5531, 73.0155) centre (-59.5464, 73.0207) ccw projected
  line L19 (-65.5531, 73.0155) -> (-65.5531, -91.7609) projected
  arc A8 (-65.5531, -91.7609) -> (-59.5464, -97.7727) centre (-59.5464, -91.766) ccw projected
  line L20 (-59.5464, -97.7727) -> (54.4883, -97.7727) projected
  arc A9 (54.4883, -97.7727) -> (60.495, -91.7609) centre (54.4883, -91.766) ccw projected
  line L21 (60.495, -91.7609) -> (60.495, 73.0155) projected
  line L22 (-58.5765, 74.3443) -> (-58.5765, 71.9392) projected
  line L23 (-58.5765, 71.9392) -> (-60.9816, 71.9392) projected
  line L24 (-60.9816, 71.9392) -> (-60.9816, 74.3443) projected
  line L25 (-60.9816, 74.3443) -> (-58.5765, 74.3443) projected
  line L26 (55.9235, -10.8013) -> (53.5184, -10.8013) projected
  line L27 (53.5184, -10.8013) -> (53.5184, -8.3961) projected
  line L28 (53.5184, -8.3961) -> (55.9235, -8.3961) projected
  line L29 (55.9235, -8.3961) -> (55.9235, -10.8013) projected
  line L30 (53.5184, 74.3443) -> (55.9235, 74.3443) projected
  line L31 (55.9235, 74.3443) -> (55.9235, 71.9392) projected
  line L32 (55.9235, 71.9392) -> (53.5184, 71.9392) projected
  line L33 (53.5184, 71.9392) -> (53.5184, 74.3443) projected
  line L34 (-60.9816, -8.3961) -> (-58.5765, -8.3961) projected
  line L35 (-58.5765, -8.3961) -> (-58.5765, -10.8013) projected
  line L36 (-58.5765, -10.8013) -> (-60.9816, -10.8013) projected
  line L37 (-60.9816, -10.8013) -> (-60.9816, -8.3961) projected
  line L38 (-58.5765, -93.5398) -> (-60.9816, -93.5398) projected
  line L39 (-60.9816, -93.5398) -> (-60.9816, -91.1346) projected
  line L40 (-60.9816, -91.1346) -> (-58.5765, -91.1346) projected
  line L41 (-58.5765, -91.1346) -> (-58.5765, -93.5398) projected
  line L42 (53.5184, -91.1346) -> (55.9235, -91.1346) projected
  line L43 (55.9235, -91.1346) -> (55.9235, -93.5398) projected
  line L44 (55.9235, -93.5398) -> (53.5184, -93.5398) projected
  line L45 (53.5184, -93.5398) -> (53.5184, -91.1346) projected
  line L46 (-60.9816, -93.5398) -> (-58.5765, -93.5398) construction
  line L47 (-58.5765, -93.5398) -> (-58.5765, -91.1346) construction
  line L48 (-58.5765, -91.1346) -> (-60.9816, -91.1346) construction
  line L49 (-60.9816, -91.1346) -> (-60.9816, -93.5398) construction
  line L50 (-60.9816, -93.5398) -> (-58.5765, -91.1346) construction
  line L51 (-58.5765, -93.5398) -> (-60.9816, -91.1346) construction
  line L52 (-60.9816, -10.8013) -> (-58.5765, -10.8013) construction
  line L53 (-58.5765, -10.8013) -> (-58.5765, -8.3961) construction
  line L54 (-58.5765, -8.3961) -> (-60.9816, -8.3961) construction
  line L55 (-60.9816, -8.3961) -> (-60.9816, -10.8013) construction
  line L56 (-60.9816, -10.8013) -> (-58.5765, -8.3961) construction
  line L57 (-58.5765, -10.8013) -> (-60.9816, -8.3961) construction
  line L58 (-60.9816, 71.9392) -> (-58.5765, 71.9392) construction
  line L59 (-58.5765, 71.9392) -> (-58.5765, 74.3443) construction
  line L60 (-58.5765, 74.3443) -> (-60.9816, 74.3443) construction
  line L61 (-60.9816, 74.3443) -> (-60.9816, 71.9392) construction
  line L62 (-60.9816, 71.9392) -> (-58.5765, 74.3443) construction
  line L63 (-58.5765, 71.9392) -> (-60.9816, 74.3443) construction
  line L64 (53.5184, -10.8013) -> (55.9235, -10.8013) construction
  line L65 (55.9235, -10.8013) -> (55.9235, -8.3961) construction
  line L66 (55.9235, -8.3961) -> (53.5184, -8.3961) construction
  line L67 (53.5184, -8.3961) -> (53.5184, -10.8013) construction
  line L68 (53.5184, -10.8013) -> (55.9235, -8.3961) construction
  line L69 (55.9235, -10.8013) -> (53.5184, -8.3961) construction
  line L70 (53.5184, -93.5398) -> (55.9235, -93.5398) construction
  line L71 (55.9235, -93.5398) -> (55.9235, -91.1346) construction
  line L72 (55.9235, -91.1346) -> (53.5184, -91.1346) construction
  line L73 (53.5184, -91.1346) -> (53.5184, -93.5398) construction
  line L74 (53.5184, -93.5398) -> (55.9235, -91.1346) construction
  line L75 (55.9235, -93.5398) -> (53.5184, -91.1346) construction
  line L76 (55.9235, -91.1346) -> (55.9235, -93.5398) construction
  line L77 (-58.5765, -10.8013) -> (-60.9816, -10.8013) construction
  line L78 (-58.5765, 71.9392) -> (-60.9816, 71.9392) construction
  line L79 (53.5184, 71.9392) -> (55.9235, 71.9392) construction
  line L80 (55.9235, 71.9392) -> (55.9235, 74.3443) construction
  line L81 (55.9235, 74.3443) -> (53.5184, 74.3443) construction
  line L82 (53.5184, 74.3443) -> (53.5184, 71.9392) construction
  line L83 (53.5184, 71.9392) -> (55.9235, 74.3443) construction
  line L84 (55.9235, 71.9392) -> (53.5184, 74.3443) construction
  line L85 (55.9235, -10.8013) -> (53.5184, -10.8013) construction
  line L86 (53.5184, -8.3961) -> (55.9235, -8.3961) construction
  line L87 (53.5184, -10.8013) -> (53.5184, -8.3961) construction
  circle A10 centre (54.721, -92.3372) radius 2.25
  circle A11 centre (54.721, -9.5987) radius 2.25
  circle A12 centre (54.721, 73.1418) radius 2.25
  circle A13 centre (-59.7791, 73.1418) radius 2.25
  circle A14 centre (-59.7791, -9.5987) radius 2.25
  circle A15 centre (-59.7791, -92.3372) radius 2.25
  point P0 (0, 0)
  dimension "d12" = 4.5
  constraints: 72 end point, 20 collinear, 12 midpoint, 12 parallel, 6 centre point, 6 coincident, 6 horizontal, 6 perpendicular, 5 equal radius
  measures "d12" diameter of A10
extrude "Extrusion5" cut sketch "Sketch5" against normal through all contours L22 L23 L24 L25 | A10 | A11 | A12 | A13 | A14 | A15
body "Solid1"
